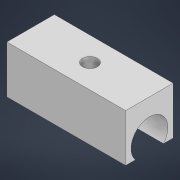
# Autodesk Inventor part: magnet dims
Saved by Autodesk Inventor 2022 (Build 260153000, 153)
## iProperties
Created: 2022-03-28
Part Number: magnet dims
Material: Generic
Document SubType Name: Modeling
Designer: Jakob Saugbjerg
Density: 1 g/cm^3
Appearance: Default
Author: Jakob Saugbjerg
Autodesk Inventor part; units mm, degrees
ref_plane "YZ Plane" through (0, 0, 0) normal (1, 0, 0) x (0, 1, 0)
ref_plane "XZ Plane" through (0, 0, 0) normal (0, 1, 0) x (-1, 0, 0)
ref_plane "XY Plane" through (0, 0, 0) normal (0, 0, 1) x (1, 0, 0)
sketch "Sketch1" plane through (0, 0, 0) normal (0, 0, 1) x (1, 0, 0)
  line L0 (-10, 4) -> (10, 4)
  line L1 (10, 4) -> (10, -4)
  line L2 (10, -4) -> (-10, -4)
  line L3 (-10, -4) -> (-10, 4)
  line L4 (-10, 4) -> (10, -4) construction
  line L5 (10, 4) -> (-10, -4) construction
  point P0 (0, 0)
  dimension "d0" = 20
  dimension "d1" = 8
  constraints: 12 end point, 2 midpoint, 2 parallel, 1 horizontal, 1 perpendicular
  measures "d0" distance of L1.end L2.end
  measures "d1" distance of L0.end L1.end
extrude "Extrusion1" add sketch "Sketch1" along normal blind 8
sketch "Sketch2" plane through (10, -4, 0) normal (1, 0, 0) x (0, 0, -1)
  line L0 (0, 0) -> (-8, 0) projected
  line L1 (-4, 0) -> (-4, 2)
  circle A0 centre (-4, 2) radius 3.1
  point P0 (0, 4)
  point P1 (-1.6315, 0)
  point P2 (-6.3685, 0)
  dimension "d4" = 2
  dimension "d5" = 6.2
  constraints: 2 end point, 1 centre point, 1 coincident, 1 midpoint, 1 vertical
  measures "d4" distance of L1.start L1.end
  measures "d5" diameter of A0
extrude "Extrusion2" cut sketch "Sketch2" against normal blind 20 contours L0 A0 picked at (-3.9802, 3.385)
sketch "Sketch3" plane through (-10, 4, 0) normal (0, 1, 0) x (1, 0, 0)
  line L0 (0, 0) -> (0, -8) projected
  line L1 (0, -4) -> (10, -4)
  circle A0 centre (10, -4) radius 1.25
  point P0 (10, 0)
  dimension "d8" = 2.5
  constraints: 2 end point, 1 centre point, 1 coincident, 1 horizontal, 1 midpoint
  measures "d8" diameter of A0
extrude "Extrusion3" cut sketch "Sketch3" against normal blind 2.5
body "Solid1"
